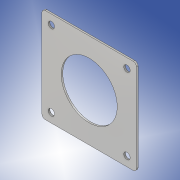
# Autodesk Inventor part: Part3
Saved by Autodesk Inventor 2017 SP1 (Build 210196100, 196)
## iProperties
Created: 2017-08-05
Part Number: Part3
Material: Aluminum 6061
Document SubType Name: Modeling
Designer: Zach
Density: 2.7 g/cm^3
Appearance: Aluminum - Polished
Author: Zach
Autodesk Inventor part; units mm, degrees
ref_plane "YZ Plane" through (0, 0, 0) normal (1, 0, 0) x (0, 1, 0)
ref_plane "XZ Plane" through (0, 0, 0) normal (0, 1, 0) x (-1, 0, 0)
ref_plane "XY Plane" through (0, 0, 0) normal (0, 0, 1) x (1, 0, 0)
sketch "Sketch1" plane through (0, 0, 0) normal (0, 0, 1) x (1, 0, 0)
  line L0 (0, 0) -> (59, 0)
  line L1 (59, 0) -> (59, 59)
  line L2 (59, 59) -> (0, 59)
  line L3 (0, 59) -> (0, 0)
  dimension "d0" = 59
  dimension "d1" = 59
  constraints: 8 end point, 2 parallel, 1 horizontal, 1 perpendicular
  measures "d0" distance of L2.end L1.end
  measures "d1" distance of L1.end L0.end
extrude "Extrusion1" add sketch "Sketch1" along normal blind 1
sketch "Sketch2" plane through (0, 0, 1) normal (0, 0, 1) x (1, 0, 0)
  circle A0 centre (29.5, 29.5) radius 17.5
  line L0 (59, 59) -> (0, 59) projected
  line L1 (0, 59) -> (0, 0) projected
  point P0 (29.5, 59)
  point P1 (0, 29.5)
  dimension "d4" = 35
  constraints: 2 midpoint, 1 centre point, 1 horizontal alignment, 1 vertical alignment
  measures "d4" diameter of A0
extrude "Extrusion2" cut sketch "Sketch2" against normal through all
sketch "Sketch3" plane through (0, 0, 1) normal (0, 0, 1) x (1, 0, 0)
  line L0 (5.9, 5.9) -> (53.1, 5.9) construction
  line L1 (53.1, 5.9) -> (53.1, 53.1) construction
  line L2 (53.1, 53.1) -> (5.9, 53.1) construction
  line L3 (5.9, 53.1) -> (5.9, 5.9) construction
  line L4 (59, 59) -> (0, 59) construction
  line L5 (0, 59) -> (0, 0) construction
  circle A0 centre (5.9, 53.1) radius 2
  circle A1 centre (53.1, 53.1) radius 2
  circle A2 centre (53.1, 5.9) radius 2
  circle A3 centre (5.9, 5.9) radius 2
  point P0 (29.5, 53.1)
  point P1 (29.5, 59)
  point P2 (53.1, 29.5)
  point P3 (0, 29.5)
  dimension "d7" = 47.2
  dimension "d8" = 47.2
  dimension "d9" = 4
  dimension "d10" = 4
  dimension "d11" = 4
  dimension "d12" = 4
  constraints: 8 end point, 4 centre point, 4 coincident, 4 midpoint, 2 parallel, 1 horizontal, 1 horizontal alignment, 1 perpendicular, 1 vertical alignment
  measures "d7" distance of L2.end L1.end
  measures "d8" distance of L1.end L0.end
  measures "d9" diameter of A0
  measures "d10" diameter of A1
  measures "d11" diameter of A2
  measures "d12" diameter of A3
extrude "Extrusion3" cut sketch "Sketch3" against normal through all
fillet "Fillet1" radius 2 4 edges at (0, 59, 0.5) (59, 59, 0.5) (59, 0, 0.5) (0, 0, 0.5)
body "Solid1"
